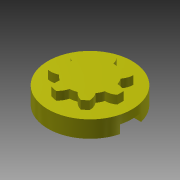
# Autodesk Inventor part: 3d-tandwiel
Saved by Autodesk Inventor 2015 (Build 190159000, 159)
## iProperties
Created: 2016-01-24
Part Number: 3d-tandwiel
Material: Generic
Document SubType Name: Modeling
Designer: david
Density: 1 g/cm^3
Appearance: Yellow
Author: david
Autodesk Inventor part; units mm, degrees
ref_plane "YZ Plane" through (0, 0, 0) normal (1, 0, 0) x (0, 1, 0)
ref_plane "XZ Plane" through (0, 0, 0) normal (0, 1, 0) x (-1, 0, 0)
ref_plane "XY Plane" through (0, 0, 0) normal (0, 0, 1) x (1, 0, 0)
sketch "Sketch1" plane through (0, 0, 0) normal (0, 0, 1) x (1, 0, 0)
  circle A0 centre (0, 0) radius 20
  dimension "d0" = 40
  constraints: 1 centre point, 1 coincident
  measures "d0" diameter of A0
extrude "Extrusion1" add sketch "Sketch1" along normal mid plane 8
sketch "Sketch2" plane through (0, 0, -4) normal (0, 0, -1) x (-1, 0, 0)
  line L0 (-20, 0) -> (20, 0) construction
  line L1 (-20, -5) -> (20, -5)
  line L2 (20, 5) -> (-20, 5)
  arc A0 (-20, 5) -> (-20, -5) centre (-20, 0) ccw
  arc A1 (20, -5) -> (20, 5) centre (20, 0) ccw
  line L3 (0, 0) -> (40, 0) construction
  dimension "d3" = 20
  dimension "d4" = 0
  dimension "d5" = 10
  constraints: 10 end point, 4 point on circle, 4 tangent, 2 centre point, 2 horizontal, 1 collinear, 1 midpoint, 1 parallel
  measures "d3" distance of L3.start L0.end
  measures "d4" distance between parallel lines of L0 L3
  measures "d5" diameter of A1
extrude "Extrusion2" cut sketch "Sketch2" against normal blind 4
sketch "Sketch6" plane through (0, 0, 4) normal (0, 0, 1) x (1, 0, 0)
  line L0 (-28, 0) -> (28, 0) projected
  arc A0 (14.5, 1.5) -> (10.0623, 3) centre (9.9997, -4.4997) ccw
  line L1 (14.5, 1.5) -> (14.5, 0)
  arc A1 (10.0623, -3) -> (14.5, -1.5) centre (9.9997, 4.4997) ccw
  line L2 (14.5, -1.5) -> (14.5, 0)
  arc A2 (7.8679, 12.2718) -> (3.9283, 9.7375) centre (9.7527, 5.0125) ccw
  line L3 (7.8679, 12.2718) -> (9.0406, 11.3366)
  line L4 (10.2133, 10.4013) -> (9.0406, 11.3366)
  arc A3 (8.6192, 5.9966) -> (10.2133, 10.4013) centre (2.7166, 10.6236) ccw
  arc A4 (-4.6889, 13.8027) -> (-5.1639, 9.1425) centre (2.1618, 10.7502) ccw
  line L5 (-4.6889, 13.8027) -> (-3.2266, 14.1365)
  line L6 (-1.7642, 14.4702) -> (-3.2266, 14.1365)
  arc A5 (0.6857, 10.4776) -> (-1.7642, 14.4702) centre (-6.6121, 8.7477) ccw
  arc A6 (-13.7149, 4.9399) -> (-10.3675, 1.663) centre (-7.057, 8.3928) ccw
  line L7 (-13.7149, 4.9399) -> (-13.064, 6.2913)
  line L8 (-12.4132, 7.6428) -> (-13.064, 6.2913)
  arc A7 (-7.7642, 7.0688) -> (-12.4132, 7.6428) centre (-10.9617, 0.2846) ccw
  arc A8 (-12.4132, -7.6428) -> (-7.7642, -7.0688) centre (-10.9617, -0.2846) ccw
  line L9 (-12.4132, -7.6428) -> (-13.064, -6.2913)
  line L10 (-13.7149, -4.9399) -> (-13.064, -6.2913)
  arc A9 (-10.3675, -1.663) -> (-13.7149, -4.9399) centre (-7.057, -8.3928) ccw
  arc A10 (-1.7642, -14.4702) -> (0.6857, -10.4776) centre (-6.6121, -8.7477) ccw
  line L11 (-1.7642, -14.4702) -> (-3.2266, -14.1365)
  line L12 (-4.6889, -13.8027) -> (-3.2266, -14.1365)
  arc A11 (-5.1639, -9.1425) -> (-4.6889, -13.8027) centre (2.1618, -10.7502) ccw
  arc A12 (10.2133, -10.4013) -> (8.6192, -5.9966) centre (2.7166, -10.6236) ccw
  line L13 (10.2133, -10.4013) -> (9.0406, -11.3366)
  line L14 (7.8679, -12.2718) -> (9.0406, -11.3366)
  arc A13 (3.9283, -9.7375) -> (7.8679, -12.2718) centre (9.7527, -5.0125) ccw
  arc A14 (10.0623, 3) -> (8.6192, 5.9966) centre (0, 0) ccw
  arc A15 (3.9283, 9.7375) -> (0.6857, 10.4776) centre (0, 0) ccw
  arc A16 (-5.1639, 9.1425) -> (-7.7642, 7.0688) centre (0, 0) ccw
  arc A17 (-10.3675, 1.663) -> (-10.3675, -1.663) centre (0, 0) ccw
  arc A18 (-7.7642, -7.0688) -> (-5.1639, -9.1425) centre (0, 0) ccw
  arc A19 (0.6857, -10.4776) -> (3.9283, -9.7375) centre (0, 0) ccw
  arc A20 (8.6192, -5.9966) -> (10.0623, -3) centre (0, 0) ccw
  dimension "d33" = 1.5
  dimension "d34" = 3
  dimension "d35" = 7.5
  dimension "d36" = 14.5
  dimension "d39" = 360
  constraints: 42 point on circle, 28 end point, 21 centre point, 3 symmetric about line, 1 coincident, 1 perpendicular, 1 point on line, 79 other
  measures "d33" distance of L1.start L1.end
  measures "d34" distance from line of A0.end L0
  measures "d35" radius of A0
  measures "d36" distance from line of A14.centre L1
extrude "Extrusion4" add sketch "Sketch6" along normal blind 4
body "Solid1"
